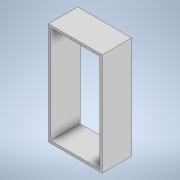
# Autodesk Inventor part: empty_room
Saved by Autodesk Inventor 2022 (Build 260153000, 153)
## iProperties
Created: 2022-10-21
Part Number: empty_room
Material: Generic
Document SubType Name: Modeling
Designer: Matthew
Density: 1 g/cm^3
Appearance: Default
Author: Matthew
Autodesk Inventor part; units mm, degrees
ref_plane "YZ Plane" through (0, 0, 0) normal (1, 0, 0) x (0, 1, 0)
ref_plane "XZ Plane" through (0, 0, 0) normal (0, 1, 0) x (-1, 0, 0)
ref_plane "XY Plane" through (0, 0, 0) normal (0, 0, 1) x (1, 0, 0)
sketch "Sketch1" plane through (0, 0, 0) normal (0, 0, 1) x (1, 0, 0)
  line L0 (0, 0) -> (254, 0)
  line L1 (254, 0) -> (254, 508)
  line L2 (254, 508) -> (0, 508)
  line L3 (0, 508) -> (0, 0)
  line L4 (-12.7, -12.7) -> (266.7, -12.7)
  line L5 (266.7, -12.7) -> (266.7, 520.7)
  line L6 (266.7, 520.7) -> (-12.7, 520.7)
  line L7 (-12.7, 520.7) -> (-12.7, -12.7)
  line L8 (-12.7, -12.7) -> (266.7, 520.7) construction
  line L9 (266.7, -12.7) -> (-12.7, 520.7) construction
  point P0 (127, 254)
  dimension "d0" = 254
  dimension "d1" = 508
  dimension "d2" = 279.4
  dimension "d3" = 533.4
  dimension "d4" = 12.7
  constraints: 20 end point, 4 parallel, 2 horizontal, 2 midpoint, 2 perpendicular
  measures "d0" distance of L2.end L1.end
  measures "d1" distance of L1.end L0.end
  measures "d2" distance of L6.end L5.end
  measures "d3" distance of L5.end L4.end
  measures "d4" distance between parallel lines of L4 L0
extrude "Extrusion1" add sketch "Sketch1" along normal blind 152.4
body "Solid1"
